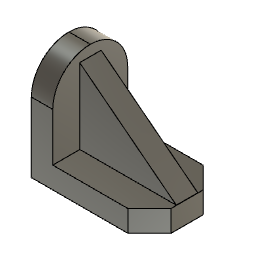
A1 (Autodesk Fusion 360 design; units mm, degrees)
Autodesk Fusion 360 part; units mm, degrees
sketch "Sketch1" plane through (0, 0, 0) normal (0, 0, 1) x (1, 0, 0)
  line L0 (33, 21) -> (-33, 21)
  line L1 (-33, 21) -> (-33, -21)
  line L2 (-33, -21) -> (33, -21)
  line L3 (33, -21) -> (33, 21)
  line L4 (33, 21) -> (-33, -21) construction
  line L5 (-33, 21) -> (33, -21) construction
  dimension "d1" = 66
  dimension "d2" = 42
  constraint horizontal L0
  constraint perpendicular L0 L1
  constraint parallel L0 L2
  constraint parallel L1 L3
  constraint coincident L4 origin
  constraint coincident L5 origin
  measures "d1" distance of L1.end L2.end
  measures "d2" distance of L0.end L1.end
extrude "Extrude1" add sketch "Sketch1" along normal blind 12 makes body 1
chamfer "Chamfer1" distance 12 angle 45 2 edges at (33, -21, 6) (33, 21, 6) on bodies 1
sketch "Sketch2" plane through (0, 0, 12) normal (0, 0, 1) x (-1, 0, 0)
  line L0 (-33, -9) -> (-21, -21)
  line L1 (-21, -21) -> (33, -21)
  line L2 (33, -21) -> (33, 21)
  line L3 (33, 21) -> (-21, 21)
  line L4 (-21, 21) -> (-33, 9)
  line L5 (-33, 9) -> (-33, -9)
  line L6 (33.0444, -20.8446) -> (21.0444, -20.8446)
  line L7 (21.0444, -20.8446) -> (21.0444, 21)
  line L8 (21.0444, 21) -> (33.0444, 21)
  line L9 (33.0444, 21) -> (33.0444, -20.8446)
  dimension "d6" = 12
  constraint horizontal L6
  constraint vertical L7
  constraint horizontal L8
  constraint vertical L9
  measures "d6" distance of L6.start L6.end
extrude "Extrude2" add sketch "Sketch2" along normal blind 48 contours L2 L3 L6 L7 L8 bodies 1
fillet "Fillet1" radius 21 2 edges at (-27.0222, -21, 60) (-27.0222, 20.8446, 60) on bodies 1
sketch "Sketch3" plane through (0, 0, 0) normal (0, 1, 0) x (1, 0, 0)
  line L0 (-21, -54.1366) -> (-21, -12.1366)
  line L1 (-21, -12.1366) -> (33, -12.1366)
  line L2 (33, -12.1366) -> (-21, -54.1366)
  dimension "d11" = 42
  dimension "d12" = 54
  constraint vertical L0
  constraint perpendicular L0 L1
  measures "d11" distance of L0.start L0.end
  measures "d12" distance of L0.end L1.end
extrude "Extrude3" add sketch "Sketch3" along normal mid plane 12 separate body makes body 2
equation "d7 = 60 mm - 12 mm"
equation "d12 = 66 mm - 12 mm"
